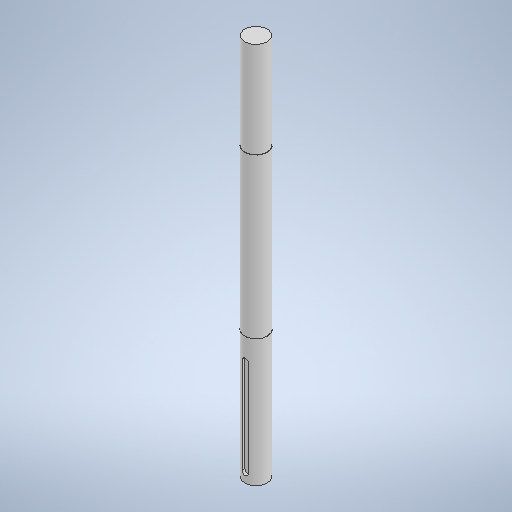
# Autodesk Inventor part: Вал ведущей шестерни
Saved by Autodesk Inventor 2026.2 (Build 302298000, 298)
## iProperties
Created: 2025-08-20
Part Number: Вал ведущей шестерни
Material: Generic
Document SubType Name: Modeling
Designer: pokla
Density: 1 g/cm^3
Appearance: Default
Author: pokla
Autodesk Inventor part; units mm, degrees
ref_plane "YZ Plane" through (0, 0, 0) normal (1, 0, 0) x (0, 1, 0)
ref_plane "XY Plane" through (0, 0, 0) normal (0, 0, 1) x (1, 0, 0)
sketch "Sketch1" plane through (0, 0, 0) normal (0, 1, 0) x (-1, 0, 0)
  line L0 (0, 0) -> (0, 600)
  line L1 (0, 0) -> (-17.5, 0)
  line L2 (-17.5, 0) -> (-17.5, 600)
  line L3 (-17.5, 600) -> (0, 600)
  line L4 (-17.5, 200) -> (-18, 200)
  line L5 (-18, 200) -> (-18, 450)
  line L6 (-18, 450) -> (-17.5, 450)
  dimension "d5" = 35
  dimension "d6" = 36
  dimension "d7" = 600
  dimension "d8" = 150
  dimension "d9" = 200
  constraints: 14 end point, 4 perpendicular, 2 point on line, 1 horizontal, 1 parallel, 1 vertical
  measures "d5" diameter of L2 L0
  measures "d6" diameter of L5 L0
  measures "d7" distance of L1.end L2.end
  measures "d8" distance between parallel lines of L3 L6
  measures "d9" distance between parallel lines of L4 L1
revolve "Revolution1" add sketch "Sketch1" angle 360 about axis through (0, 0, 0) along (0, 0, 1)
ref_plane "Work Plane2" through (0, -17.5, 525) normal (0, 1, 0) x (-1, 0, 0)
sketch "Sketch2" plane through (0, -17.5, 525) normal (0, 1, 0) x (-1, 0, 0)
  line L0 (0, -360) -> (0, -510) construction
  line L1 (-5, -360) -> (-5, -510)
  line L2 (5, -510) -> (5, -360)
  arc A0 (5, -360) -> (-5, -360) centre (0, -360) ccw
  arc A1 (-5, -510) -> (5, -510) centre (0, -510) ccw
  point P0 (0, -525)
  point P1 (0, -435)
  point P2 (0, -515)
  dimension "d10" = 10
  dimension "d11" = 150
  dimension "d12" = 10
  constraints: 8 end point, 5 point on circle, 4 tangent, 2 centre point, 1 midpoint, 1 parallel, 1 vertical, 1 vertical alignment
  measures "d10" distance between parallel lines of L1 L2
  measures "d11" distance of L0.start L0.end
  measures "d12" distance of point (0, -525) point (0, -515)
extrude "Extrusion1" cut sketch "Sketch2" along normal blind 5
body "Solid1"
